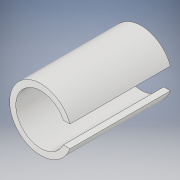
# Autodesk Inventor part: coupler
Saved by Autodesk Inventor 2017 (Build 210142000, 142)
## iProperties
Created: 2018-11-30
Part Number: coupler
Material: Acetal Resin, White
Document SubType Name: Modeling
Designer: ddeboer
Density: 1.425 g/cm^3
Appearance: Smooth - White
Author: ddeboer
Autodesk Inventor part; units mm, degrees
ref_plane "YZ Plane" through (0, 0, 0) normal (1, 0, 0) x (0, 1, 0)
ref_plane "XZ Plane" through (0, 0, 0) normal (0, 1, 0) x (-1, 0, 0)
ref_plane "XY Plane" through (0, 0, 0) normal (0, 0, 1) x (1, 0, 0)
sketch "Sketch1" plane through (0, 0, 0) normal (0, 0, 1) x (1, 0, 0)
  circle A0 centre (0, 0) radius 16.713
  circle A1 centre (0, 0) radius 13.4
  dimension "d0" = 33.426
  dimension "d1" = 26.8
  constraints: 2 centre point, 2 coincident
  measures "d0" diameter of A0
  measures "d1" diameter of A1
extrude "Extrusion1" add sketch "Sketch1" along normal blind 53.9
sketch "Sketch4" plane through (0, 0, 53.9) normal (0, 0, 1) x (1, 0, 0)
  line L0 (0, -5.75) -> (20, -5.75)
  line L1 (20, -5.75) -> (20, 5.75)
  line L2 (20, 5.75) -> (0, 5.75)
  line L3 (0, 5.75) -> (0, -5.75)
  point P0 (0, 0)
  point P1 (0, 0)
  dimension "d9" = 20
  dimension "d10" = 11.5
  constraints: 8 end point, 2 parallel, 1 coincident, 1 horizontal, 1 midpoint, 1 perpendicular
  measures "d9" distance of L2.end L1.end
  measures "d10" distance of L1.end L0.end
extrude "Extrusion4" cut sketch "Sketch4" against normal up to next
body "Solid1"
